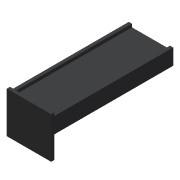
# Autodesk Inventor part: slidelat
Saved by Autodesk Inventor 2022 Beta2 (Build 260130000, 130) ContinuousBuild 0
## iProperties
Shininess: 64.0
Length Units: 11272
Angle Units: 11279
Time Units: 11290
Mass Units: 11286
Length Display Precision: 3
Angle Display Precision: 2
Created: 2002-04-25
Part Number: slidelat
Document SubType Name: Modeling
Designer: Administrator
Stock Number: slidelat
Density: 1 g/cm^3
Material: Generic
Appearance: Generic
Density: 0.0
Volumn: 0.0
Area: 0.0
PropertySet Name: Model Information
Control State: 0
Master: False
Checked Out: False
Author: Administrator
Autodesk Inventor part; units mm, degrees
ref_plane "YZ Plane" through (0, 0, 0) normal (1, 0, 0) x (0, 1, 0)
ref_plane "XZ Plane" through (0, 0, 0) normal (0, 1, 0) x (-1, 0, 0)
sketch "Sketch1" plane through (0, 0, 0) normal (0, 0, 1) x (1, 0, 0)
  line L0 (-28.5226, 14.562) -> (-28.5226, 1.862)
  line L1 (-28.5226, 1.862) -> (-25.9826, 1.862)
  line L2 (-25.9826, 1.862) -> (-25.9826, 6.942)
  line L3 (-25.9826, 6.942) -> (4.4974, 6.942)
  line L4 (4.4974, 6.942) -> (4.4974, 1.862)
  line L5 (4.4974, 1.862) -> (7.0374, 1.862)
  line L6 (7.0374, 1.862) -> (7.0374, 14.562)
  line L7 (7.0374, 14.562) -> (4.4974, 14.562)
  line L8 (4.4974, 14.562) -> (4.4974, 12.022)
  line L9 (4.4974, 12.022) -> (-25.9826, 12.022)
  line L10 (-25.9826, 12.022) -> (-25.9826, 14.562)
  line L11 (-25.9826, 14.562) -> (-28.5226, 14.562)
  dimension "d0" = 35.56
  dimension "d1" = 2.54
  dimension "d2" = 12.7
  dimension "d3" = 5.08
  dimension "d4" = 2.54
  dimension "d5" = 2.54
  constraints: 24 end point, 9 parallel, 5 collinear, 1 perpendicular, 1 vertical
  measures "d0" distance of L5.end L0.end
  measures "d1" distance of L4.end L5.end
  measures "d2" distance of L5.end L6.end
  measures "d3" distance of L1.end L2.end
  measures "d4" distance of L6.end L7.end
  measures "d5" distance of L9.end L10.end
extrude "Extrusion1" add sketch "Sketch1" along normal blind 95.25
sketch "Sketch2" plane through (-25.9826, 6.942, 0) normal (0, -1, 0) x (1, 0, 0)
  line L0 (30.48, 95.25) -> (0, 95.25) projected
  line L1 (0, 69.85) -> (2.54, 69.85)
  line L2 (2.54, 69.85) -> (2.54, 68.326)
  line L3 (2.54, 68.326) -> (0, 68.326)
  line L4 (0, 68.326) -> (0, 69.85)
  line L5 (0, 0) -> (0, 95.25) projected
  dimension "d8" = 1.524
  dimension "d9" = 2.54
  dimension "d10" = 25.4
  constraints: 8 end point, 2 parallel, 1 collinear, 1 horizontal, 1 perpendicular
  measures "d8" distance of L3.end L1.start
  measures "d9" distance of L1.start L1.end
  measures "d10" distance between parallel lines of L1 L0
extrude "Extrusion2" add sketch "Sketch2" along normal up to surface (5.08 mm away)
pattern_linear "Rectangular Pattern1" count 10 spacing 5.08 along (0, 0, -1) of "Extrusion2"
sketch "Sketch3" plane through (-25.9826, 6.942, 0) normal (0, -1, 0) x (1, 0, 0)
  line L0 (0, 49.53) -> (2.54, 49.53) projected
  line L1 (2.54, 49.53) -> (2.54, 48.006) projected
  line L2 (2.54, 48.006) -> (0, 48.006) projected
  line L3 (0, 44.45) -> (0, 48.006) projected
  line L4 (0, 44.45) -> (2.54, 44.45) projected
  line L5 (2.54, 44.45) -> (2.54, 42.926) projected
  line L6 (2.54, 42.926) -> (0, 42.926) projected
  line L7 (0, 0) -> (0, 42.926) projected
  line L8 (0, 0) -> (30.48, 0) projected
  line L9 (30.48, 0) -> (30.48, 95.25) projected
  line L10 (30.48, 95.25) -> (0, 95.25) projected
  line L11 (0, 69.85) -> (0, 95.25) projected
  line L12 (0, 69.85) -> (2.54, 69.85) projected
  line L13 (2.54, 69.85) -> (2.54, 68.326) projected
  line L14 (2.54, 68.326) -> (0, 68.326) projected
  line L15 (0, 64.77) -> (0, 68.326) projected
  line L16 (0, 64.77) -> (2.54, 64.77) projected
  line L17 (2.54, 64.77) -> (2.54, 63.246) projected
  line L18 (2.54, 63.246) -> (0, 63.246) projected
  line L19 (0, 59.69) -> (0, 63.246) projected
  line L20 (0, 59.69) -> (2.54, 59.69) projected
  line L21 (2.54, 59.69) -> (2.54, 58.166) projected
  line L22 (2.54, 58.166) -> (0, 58.166) projected
  line L23 (0, 54.61) -> (0, 58.166) projected
  line L24 (0, 54.61) -> (2.54, 54.61) projected
  line L25 (2.54, 54.61) -> (2.54, 53.086) projected
  line L26 (2.54, 53.086) -> (0, 53.086) projected
  line L27 (0, 49.53) -> (0, 53.086) projected
  line L28 (15.24, 80.1212) -> (15.24, 49.6412)
  circle A0 centre (15.24, 64.8812) radius 15.24 construction
  line L29 (30.48, 0) -> (30.48, 95.25) projected
  line L30 (0, 69.85) -> (0, 95.25) projected
  constraints: 2 end point, 2 point on circle, 2 tangent, 1 centre point, 1 midpoint, 1 parallel
ref_plane "Work Plane1" through (-10.7426, 6.942, 80.1212) normal (-1, 0, 0) x (0, -1, 0)
sketch "Sketch4" plane through (-25.9826, 6.942, 0) normal (0, -1, 0) x (1, 0, 0)
  line L0 (0, 0) -> (0, 22.606) projected
  line L1 (0, 0) -> (30.48, 0) projected
  line L2 (0, 0) -> (5.8186, 0)
  line L3 (0, 5.08) -> (4.318, 5.08)
  line L4 (4.318, 5.08) -> (4.318, 0)
  dimension "d17" = 5.08
  dimension "d18" = 4.318
  constraints: 6 end point, 3 point on line, 1 parallel, 1 perpendicular
  measures "d17" distance of L3.end L4.end
  measures "d18" distance of L3.start L3.end
extrude "Extrusion3" add sketch "Sketch4" along normal up to surface (5.08 mm away)
mirror "Mirror1" about plane through (-10.7426, 6.942, 80.1212) normal (-1, 0, 0) of "Extrusion2", "Rectangular Pattern1"
mirror "Mirror2" about plane through (-10.7426, 6.942, 80.1212) normal (-1, 0, 0) of "Extrusion3"
sketch "Sketch5" plane through (0, 0, 95.25) normal (0, 0, 1) x (1, 0, 0)
  line L0 (-28.5226, 14.562) -> (-25.9826, 14.562) projected
  line L1 (-28.5226, 1.862) -> (-28.5226, 14.562) projected
  line L2 (-25.9826, 1.862) -> (-28.5226, 1.862) projected
  line L3 (-25.9826, 6.942) -> (-25.9826, 1.862) projected
  line L4 (4.4974, 6.942) -> (-25.9826, 6.942) projected
  line L5 (4.4974, 1.862) -> (4.4974, 6.942) projected
  line L6 (7.0374, 1.862) -> (4.4974, 1.862) projected
  line L7 (7.0374, 14.562) -> (7.0374, 1.862) projected
  line L8 (4.4974, 14.562) -> (7.0374, 14.562) projected
  line L9 (4.4974, 12.022) -> (4.4974, 14.562) projected
  line L10 (-25.9826, 12.022) -> (4.4974, 12.022) projected
  line L11 (-25.9826, 14.562) -> (-25.9826, 12.022) projected
  line L12 (-28.5226, 17.102) -> (7.0374, 17.102)
  line L13 (7.0374, 17.102) -> (7.0374, -15.918)
  line L14 (7.0374, -15.918) -> (-28.5226, -15.918)
  line L15 (-28.5226, -15.918) -> (-28.5226, 17.102)
  dimension "d21" = 33.02
  dimension "d22" = 17.78
  constraints: 8 end point, 2 collinear, 2 parallel, 1 horizontal, 1 perpendicular
  measures "d21" distance of L14.end L12.start
  measures "d22" distance between parallel lines of L6 L14
extrude "Extrusion4" add sketch "Sketch5" along normal blind 2.54
body "Solid1"
